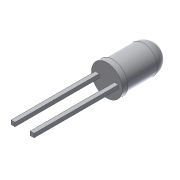
# Autodesk Inventor part: P02 - LED 5mm
Saved by Autodesk Inventor 2016 (Build 200138000, 138)
## iProperties
Created: 2016-12-26
Part Number: P02 - LED 5mm
Material: ABS Plastic
Document SubType Name: Modeling
Designer: Fernando
Stock Number: 0
Mass: 0.189926 g
Surface Area: 2.54824 cm^2
Volume: 0.179175 cm^3
Density: 1.06 g/cm^3
Appearance: Smooth - White
SurfaceArea_m2: 0
Author: Fernando
Autodesk Inventor part; units mm, degrees
ref_plane "YZ Plane" through (0, 0, 0) normal (1, 0, 0) x (0, 1, 0)
ref_plane "XZ Plane" through (0, 0, 0) normal (0, 1, 0) x (-1, 0, 0)
ref_plane "XY Plane" through (0, 0, 0) normal (0, 0, 1) x (1, 0, 0)
sketch "Sketch2" plane through (0, 0, 0) normal (0, 0, 1) x (1, 0, 0)
  line L0 (0, 0) -> (0, 6.5)
  line L1 (0, 6.5) -> (-2.5, 6.5) construction
  line L2 (-2.5, 6.5) -> (-2.5, 1)
  line L3 (-2.5, 1) -> (-2.75, 1)
  line L4 (-2.75, 1) -> (-2.75, 0)
  line L5 (-2.75, 0) -> (0, 0)
  arc A0 (0, 9) -> (-2.5, 6.5) centre (0, 6.5) ccw
  line L6 (0, 9) -> (0, 6.5)
  dimension "d11" = 5
  dimension "d12" = 5.5
  dimension "d13" = 5.5
  dimension "d14" = 1
  constraints: 14 end point, 5 perpendicular, 2 point on circle, 2 vertical, 1 centre point, 1 coincident
  measures "d11" diameter of L2 L0
  measures "d12" diameter of L4 L0
  measures "d13" distance of L1.end L2.end
  measures "d14" distance of L3.end L4.end
revolve "Revolution1" add sketch "Sketch2" angle 360 about axis through (0, 0, 0) along (0, 1, 0)
sketch "Sketch3" plane through (0, 0, 0) normal (0, -1, 0) x (1, 0, 0)
  line L0 (-2.05, -0.35) -> (-1.35, -0.35)
  line L1 (-1.35, -0.35) -> (-1.35, 0.35)
  line L2 (-1.35, 0.35) -> (-2.05, 0.35)
  line L3 (-2.05, 0.35) -> (-2.05, -0.35)
  line L4 (-2.05, -0.35) -> (-1.35, 0.35) construction
  line L5 (-1.35, -0.35) -> (-2.05, 0.35) construction
  line L6 (1.35, -0.35) -> (2.05, -0.35)
  line L7 (2.05, -0.35) -> (2.05, 0.35)
  line L8 (2.05, 0.35) -> (1.35, 0.35)
  line L9 (1.35, 0.35) -> (1.35, -0.35)
  line L10 (1.35, -0.35) -> (2.05, 0.35) construction
  line L11 (2.05, -0.35) -> (1.35, 0.35) construction
  point P0 (0, 0)
  point P1 (-1.7, 0)
  point P2 (1.7, 0)
  point P3 (1.7, 0)
  dimension "d16" = 0.7
  dimension "d17" = 1.7
  dimension "d18" = 1.7
  constraints: 24 end point, 5 midpoint, 4 parallel, 3 equal length, 3 horizontal alignment, 2 horizontal, 2 perpendicular, 1 point on line
  measures "d16" distance of L0.end L1.end
  measures "d17" distance of point (0, 0) point (-1.7, 0)
  measures "d18" distance of point (1.7, 0) point (0, 0)
extrude "Extrusion2" add sketch "Sketch3" along normal blind 15
body "Solid2"
